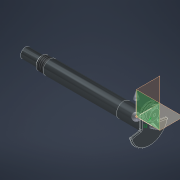
# Autodesk Inventor part: P015-Vilbrequin
Saved by Autodesk Inventor 2021.3 (Build 253353000, 353)
## iProperties
Company: HES-SO
Created: 2022-04-01
Part Number: P015-Vilbrequin
Material: Iron, Gray
Document SubType Name: Modeling
Designer: Rémi & Elise
Density: 7.15 g/cm^3
Appearance: Iron Gray
Mass: 70.8788 g
Surface Area: 48.6413 cm^2
Volume: 9.91312 cm^3
Author: Rémi & Elise
Title: P015 - Vilebrequin
Autodesk Inventor part; units mm, degrees
ref_plane "YZ Plane" through (0, 0, 0) normal (1, 0, 0) x (0, 1, 0)
ref_plane "XZ Plane" through (0, 0, 0) normal (0, 1, 0) x (-1, 0, 0)
ref_plane "XY Plane" through (0, 0, 0) normal (0, 0, 1) x (1, 0, 0)
sketch "Sketch2" plane through (0, 0, 0) normal (1, 0, 0) x (0, 1, 0)
  arc A0 (-22.6506, -3.9939) -> (22.6506, -3.9939) centre (0, 0) ccw
  line L0 (-22.6506, -3.9939) -> (-10, -1.7633)
  line L1 (-10, -1.7633) -> (-10, 13)
  line L2 (22.6506, -3.9939) -> (10, -1.7633)
  line L3 (10, -1.7633) -> (10, 13)
  arc A1 (10, 13) -> (-10, 13) centre (0, 13) ccw
  dimension "d1" = 20
  dimension "d3" = 23
  dimension "d54" = 100
  dimension "d55" = 100
  dimension "d57" = 13
  constraints: 8 end point, 4 point on circle, 2 centre point, 2 horizontal alignment, 2 point on line, 1 coincident, 1 vertical, 1 vertical alignment
  measures "d1" distance between parallel lines of L3 L1
  measures "d3" radius of A0
  measures "d54" angle of L2 L3
  measures "d55" angle of L1 L0
  measures "d57" distance of point (0, 0) A1.centre
extrude "Extrusion1" add sketch "Sketch2" along normal blind 3
sketch "Sketch10" plane through (0, 0, 0) normal (-1, 0, 0) x (0, 0, 1)
  circle A0 centre (0, 0) radius 6
  dimension "d25" = 12
  constraints: 1 centre point, 1 coincident
  measures "d25" diameter of A0
sketch "Sketch11" plane through (3, 0, 0) normal (1, 0, 0) x (0, 0, -1)
  circle A0 centre (-13, 0) radius 6
  circle A1 centre (-13, 0) radius 8
  arc A2 (3.9939, -22.6506) -> (3.9939, 22.6506) centre (0, 0) ccw projected
  line L0 (3.9939, 22.6506) -> (1.7633, 10) projected
  line L1 (1.7633, 10) -> (-13, 10) projected
  arc A3 (-13, 10) -> (-13, -10) centre (-13, 0) ccw projected
  line L2 (-13, -10) -> (1.7633, -10) projected
  line L3 (1.7633, -10) -> (3.9939, -22.6506) projected
  dimension "d29" = 12
  dimension "d32" = 2
  constraints: 2 centre point, 2 coincident, 1 horizontal alignment
  measures "d29" diameter of A0
  measures "d32" radial gap between concentric circles of A1 A0
extrude "Extrusion9" add sketch "Sketch11" along normal blind 6 contours A0
extrude "Extrusion10" add sketch "Sketch11" along normal blind 2 contours A1
sketch "Sketch12" plane through (9, 0, 13) normal (1, 0, 0) x (0, 0, -1)
  circle A0 centre (0, 0) radius 6 construction
  point P0 (13, 0)
  constraints: 1 coincident
hole "Hole2" at (9, 0, 13) direction (-1, 0, 0) diameter 3.242 depth 6 tip angle 118 thread size "M4x0.7" class "6H" standard "ISO Metric profile"
fillet "Fillet3" radius 1 16 edges at (3, 0, -23) (3, 16.3253, -2.8786) (3, 10, 5.6184) (3, 0, 23) (3, -10, 5.6184) (3, -16.3253, -2.8786) (0, 0, -23) (0, -16.3253, -2.8786) (0, -10, 5.6184) (0, 0, 23) (0, 10, 5.6184) (0, 16.3253, -2.8786) (1.5, -10, -1.7633) (1.5, -22.6506, -3.9939) (1.5, 10, -1.7633) (1.5, 22.6506, -3.9939)
sketch "Sketch13" plane through (0, 0, 0) normal (0, 1, 0) x (-1, 0, 0)
  line L0 (178.32, 0) -> (-29.72, 0) projected
  line L1 (0, 0) -> (0, 9)
  line L2 (143.6, 6) -> (143.6, 0)
  line L3 (143.6, 0) -> (0, 0)
  line L4 (0, -4.8011) -> (0, -22) projected
  line L5 (143.6, 6) -> (123.6, 6)
  line L6 (123.6, 6) -> (123.6, 8)
  line L7 (123.6, 8) -> (113.6, 8)
  line L8 (113.6, 8) -> (113.6, 8.5)
  line L9 (113.6, 8.5) -> (23.6, 8.5)
  line L10 (23.6, 8.5) -> (23.6, 9)
  line L11 (23.6, 9) -> (0, 9)
  point P0 (0, 8.5)
  dimension "d62" = 12
  dimension "d63" = 16
  dimension "d64" = 17
  dimension "d65" = 18
  dimension "d66" = 20
  dimension "d67" = 10
  dimension "d68" = 90
  dimension "d76" = 23.6
  constraints: 20 end point, 7 perpendicular, 3 point on line, 1 horizontal, 1 vertical
  measures "d62" diameter of L5 L0
  measures "d63" diameter of L7 L0
  measures "d64" diameter of L9 L0
  measures "d65" diameter of L11 L0
  measures "d66" distance of L2.start L5.end
  measures "d67" distance of L6.end L7.end
  measures "d68" distance of L8.end L9.end
  measures "d76" distance of L10.end L1.end
revolve "Revolution1" add sketch "Sketch13" angle 360 about axis through (-10, 0, 0) along (1, 0, 0)
thread "Thread1" size "M16x2" class "6g" standard "ISO Metric profile" full length
chamfer "Chamfer2" distance 1 angle 45 1 edges at (-123.6, 0, -8)
equation "\"d55\" = d54"
body "Solid1"
